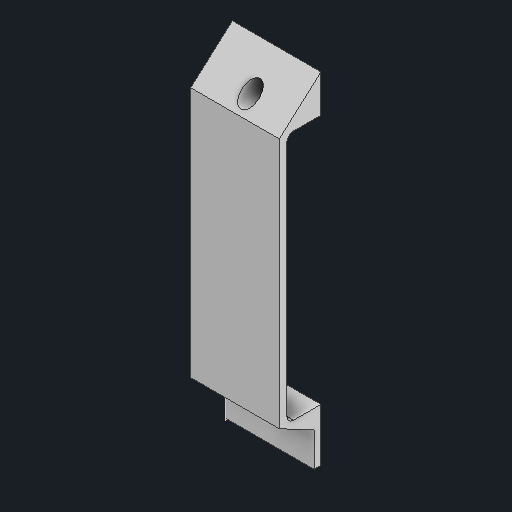
# Autodesk Inventor part: NNfront-huta
Saved by Autodesk Inventor 2026.1 (Build 301233020, 233B)
## iProperties
Created: 2026-03-18
Part Number: NNfront-huta
Material: 一般
Document SubType Name: Modeling
Designer: kamada
Density: 1 g/cm^3
Appearance: 既定
Author: kamada
Autodesk Inventor part; units mm, degrees
ref_plane "YZ Plane" through (0, 0, 0) normal (1, 0, 0) x (0, 1, 0)
ref_plane "XZ Plane" through (0, 0, 0) normal (0, 1, 0) x (-1, 0, 0)
sketch "スケッチ1" plane through (0, 0, 0) normal (0, 0, 1) x (1, 0, 0)
  ellipse E0 centre (-0.0006, 2.529) end of major axis (-0.0006, 5.5657) minor radius 3.0367 (2.9994, 3) -> (1.7646, 5) ccw projected
  line L0 (1.7646, 5) -> (-1.7658, 5) projected
  ellipse E1 centre (-0.0006, 2.529) end of major axis (-0.0006, 5.5657) minor radius 3.0367 (-1.7658, 5) -> (-3.0006, 3) ccw projected
  arc A0 (-6.0006, 0) -> (-3.0006, 3) centre (-6.0006, 3) ccw projected
  line L1 (-6.0006, 0) -> (-13.25, 0) projected
  line L2 (-13.25, -5) -> (-13.25, 0) projected
  line L3 (-13.25, -5) -> (13.25, -5) projected
  line L4 (13.25, 0) -> (13.25, -5) projected
  line L5 (13.25, 0) -> (5.9994, 0) projected
  ellipse E2 centre (5.9994, 3) end of major axis (8.9994, 3) minor radius 3 (2.9994, 3) -> (5.9994, 0) ccw projected
  circle A1 centre (-0.0006, 2.529) radius 1 projected
  point P0 (0, 0)
  constraints: 3 other
ref_plane "作業平面1" through (13.25, -5, 2) normal (0, 0, 1) x (1, 0, 0)
extrude "押し出し1" add sketch "スケッチ1" along normal up to surface (2 mm away)
sketch "スケッチ2" plane through (-13.25, -5, 2) normal (0, 0, 1) x (1, 0, 0)
  circle A0 centre (13.2494, 7.529) radius 1 projected
  line L0 (19.2494, 5) -> (26.5, 5) projected
  ellipse E0 centre (19.2494, 8) end of major axis (16.2494, 8) minor radius 3 (16.2494, 8) -> (19.2494, 5) ccw projected
  ellipse E1 centre (13.2494, 7.529) end of major axis (13.2494, 10.5657) minor radius 3.0367 (16.2494, 8) -> (15.0146, 10) ccw projected
  line L1 (11.4842, 10) -> (15.0146, 10) projected
  ellipse E2 centre (13.2494, 7.529) end of major axis (13.2494, 10.5657) minor radius 3.0367 (11.4842, 10) -> (10.2494, 8) ccw projected
  arc A1 (7.2494, 5) -> (10.2494, 8) centre (7.2494, 8) ccw projected
  line L2 (0, 5) -> (7.2494, 5) projected
  line L3 (0, 0) -> (0, 5) projected
  line L4 (26.5, 0) -> (0, 0) projected
  line L5 (26.5, 5) -> (26.5, 0) projected
  line L6 (26.5, 0) -> (26.25, 0)
  line L7 (26.25, 0) -> (26.25, 5)
  line L8 (26.25, 5) -> (26.5, 5)
  line L9 (26.5, 5) -> (26.5, 0)
  line L10 (0, 0) -> (0.25, 0)
  line L11 (0.25, 0) -> (0.25, 5)
  line L12 (0.25, 5) -> (0, 5)
  line L13 (0, 5) -> (0, 0)
  point P0 (13.25, 5)
  point P1 (0.25, 0)
  point P2 (26.25, 0)
  dimension "d2" = 0.25
  dimension "d3" = 0.25
  constraints: 16 end point, 4 parallel, 2 horizontal, 2 perpendicular, 2 point on line, 3 other
  measures "d2" distance of L7.end L8.end
  measures "d3" distance of L12.end L11.end
extrude "押し出し2" cut sketch "スケッチ2" against normal blind 10 contours L0 L5 L4 L7 | L4 L3 L2 L11
ref_plane "作業平面2" through (-13, 0, 2) normal (-1, 0, 0) x (0, -1, 0)
sketch "スケッチ3" plane through (-13, 0, 2) normal (-1, 0, 0) x (0, -1, 0)
  line L0 (-95, -2) -> (-84.0931, 10.235) projected
  line L1 (-84.0931, 10.235) -> (-10.4333, 10.235) projected
  line L2 (-10.4333, 10.235) -> (-5, 0) projected
  line L3 (-5, 0) -> (5, 0) projected
  line L4 (5, 0) -> (5, -3) projected
  line L5 (-95, -3) -> (5, -3) projected
  line L6 (-95, -2) -> (-95, -3) projected
  line L7 (-11, -11.065) -> (-11, 7.535) projected
  line L8 (-11, 7.535) -> (-84.5, 7.535) projected
  line L9 (-5, -2) -> (-5, 0) projected
  line L10 (-5, -2) -> (-10.5, -2)
  line L11 (-10.5, -2) -> (-10.5, 8.035)
  line L12 (-10.5, 8.035) -> (-12.7452, 8.035)
  line L13 (-12.7452, 8.035) -> (-84.6975, 8.035)
  line L14 (-85, -6.5) -> (-85, -5) projected
  line L15 (-85, -2) -> (-85, -5) projected
  line L16 (-85, -2) -> (-85, 8.035)
  line L17 (-85, 8.035) -> (-84.5, 8.035)
  line L18 (-85, -2) -> (-95, -2)
  point P0 (0, -2)
  dimension "d6" = 0.5
  dimension "d7" = 0.5
  constraints: 14 end point, 2 horizontal, 2 perpendicular, 1 parallel, 1 point on line, 1 vertical
  measures "d6" distance between parallel lines of L11 L7
  measures "d7" distance between parallel lines of L12 L8
extrude "押し出し3" add sketch "スケッチ3" against normal up to surface (26 mm away) contours L0 L1 L2 L9 L10 L11 L12 L13 L17 L16 L18
sketch "スケッチ4" plane through (0, 0, 0) normal (0, 0, -1) x (-1, 0, 0)
  circle A0 centre (0.0006, 2.529) radius 1 projected
  line L0 (13, -5) -> (13, 0) projected
  line L1 (6.0006, 0) -> (13, 0) projected
  arc A1 (3.0006, 3) -> (6.0006, 0) centre (6.0006, 3) ccw projected
  ellipse E0 centre (0.0006, 2.529) end of major axis (0.0006, 5.5657) minor radius 3.0367 (3.0006, 3) -> (1.7658, 5) ccw projected
  line L2 (13, 5) -> (1.7658, 5) projected
  line L3 (13, 10.5) -> (13, 5) projected
  line L4 (13, 10.5) -> (-13, 10.5) projected
  line L5 (-13, 5) -> (-13, 10.5) projected
  line L6 (-1.7646, 5) -> (-13, 5) projected
  ellipse E1 centre (0.0006, 2.529) end of major axis (0.0006, 5.5657) minor radius 3.0367 (-1.7646, 5) -> (-2.9994, 3) ccw projected
  ellipse E2 centre (-5.9994, 3) end of major axis (-2.9994, 3) minor radius 3 (-5.9994, 0) -> (-2.9994, 3) ccw projected
  line L7 (-13, 0) -> (-5.9994, 0) projected
  line L8 (-13, 0) -> (-13, -5) projected
  line L9 (13, -5) -> (-13, -5) projected
  line L10 (-13, 0) -> (-13, 5)
  line L11 (13, 5) -> (13, 0)
  point P0 (0, 0)
  constraints: 4 end point, 1 perpendicular, 1 vertical, 3 other
extrude "押し出し4" add sketch "スケッチ4" against normal up to surface (2 mm away) contours L1 A1 E0 L2 L11 | L10 L6 E1 E2 L7
sketch "スケッチ5" plane through (-13, 10.4333, 12.235) normal (0, 0, 1) x (1, 0, 0)
  circle A0 centre (13.7123, 77.0667) radius 1 projected
  circle A1 centre (13.7123, 77.0667) radius 2.5
  point P0 (13, -10.4333)
  dimension "d12" = 5
  constraints: 1 centre point, 1 coincident
  measures "d12" diameter of A1
extrude "押し出し5" cut sketch "スケッチ5" against normal blind 13 contours A0
sketch "スケッチ6" plane through (-13, 10.4333, 12.235) normal (0, 0, 1) x (1, 0, 0)
  circle A0 centre (13.7123, 77.0667) radius 1 projected
  circle A1 centre (13.7123, 77.0667) radius 2.5
  point P0 (13, -10.4333)
  dimension "d15" = 5
  constraints: 1 centre point, 1 coincident
  measures "d15" diameter of A1
extrude "押し出し6" cut sketch "スケッチ6" against normal blind 11 contours A0 | A1
sketch "スケッチ7" plane through (-13, 85, 0) normal (0, -1, 0) x (1, 0, 0)
  line L0 (26, 10.035) -> (26, 0) projected
  line L1 (13.7123, 10.035) -> (26, 10.035) projected
  line L2 (13.7123, 10.035) -> (13.7123, 1.235) projected
  line L3 (0, 10.035) -> (13.7123, 10.035) projected
  line L4 (0, 0) -> (0, 10.035) projected
  line L5 (0, 0) -> (26, 0) projected
  point P0 (13, 0)
extrude "押し出し7" add sketch "スケッチ7" along normal blind 1
fillet "フィレット1" radius 2 2 edges at (0, 10.5, 10.035) (0, 84, 10.035)
equation "\"d7\" = d6"
